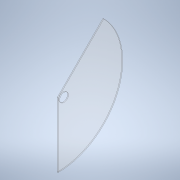
# Autodesk Inventor part: Shooter side panel
Saved by Autodesk Inventor 2021 (Build 250183000, 183)
## iProperties
Created: 2021-02-04
Part Number: Shooter side panel
Material: Polycarbonate, Clear
Document SubType Name: Modeling
Designer: aidan
Density: 1.2 g/cm^3
Appearance: Polycarbonate - Clear
Author: aidan
Autodesk Inventor part; units mm, degrees
ref_plane "YZ Plane" through (0, 0, 0) normal (1, 0, 0) x (0, 1, 0)
ref_plane "XZ Plane" through (0, 0, 0) normal (0, 1, 0) x (-1, 0, 0)
ref_plane "XY Plane" through (0, 0, 0) normal (0, 0, 1) x (1, 0, 0)
sketch "Sketch1" plane through (0, 0, 0) normal (1, 0, 0) x (0, 1, 0)
  line L0 (0, 0) -> (148.1742, -148.1742)
  line L1 (0, 0) -> (-209.55, 0)
  arc A0 (-209.55, 0) -> (148.1742, -148.1742) centre (0, 0) ccw
  circle A1 centre (-7.8908, -19.05) radius 14.2875
  line L2 (0, 0) -> (-7.8908, -19.05) construction
  circle A2 centre (-7.8908, -19.05) radius 25.4 construction
  arc A3 (-196.85, 0) -> (139.194, -139.194) centre (0, 0) ccw construction
  arc A4 (-209.55, 0) -> (148.1742, -148.1742) centre (0, 0) ccw construction
  arc A5 (-184.15, 0) -> (130.2137, -130.2137) centre (0, 0) ccw construction
  arc A6 (-184.15, 0) -> (-209.55, 0) centre (-196.85, 0) ccw construction
  arc A7 (148.1742, -148.1742) -> (130.2137, -130.2137) centre (139.194, -139.194) ccw construction
  dimension "d0" = 135
  dimension "d1" = 67.5
  dimension "d2" = 28.575
  dimension "d3" = 19.05
  dimension "d4" = 50.8
  dimension "d5" = 209.55
  dimension "d8" = 12.7
  constraints: 12 point on circle, 8 centre point, 6 end point, 5 tangent, 3 coincident, 3 point on line, 1 equal length, 1 horizontal
  measures "d0" angle of L1 L0
  measures "d1" angle of L0 L2
  measures "d2" diameter of A1
  measures "d3" distance from line of L1 L2.end
  measures "d4" diameter of A2
  measures "d5" radius of A0
  measures "d8" radial gap between concentric circles of A0 A3
extrude "Extrusion1" add sketch "Sketch1" along normal blind 2.9972
body "Solid1"
